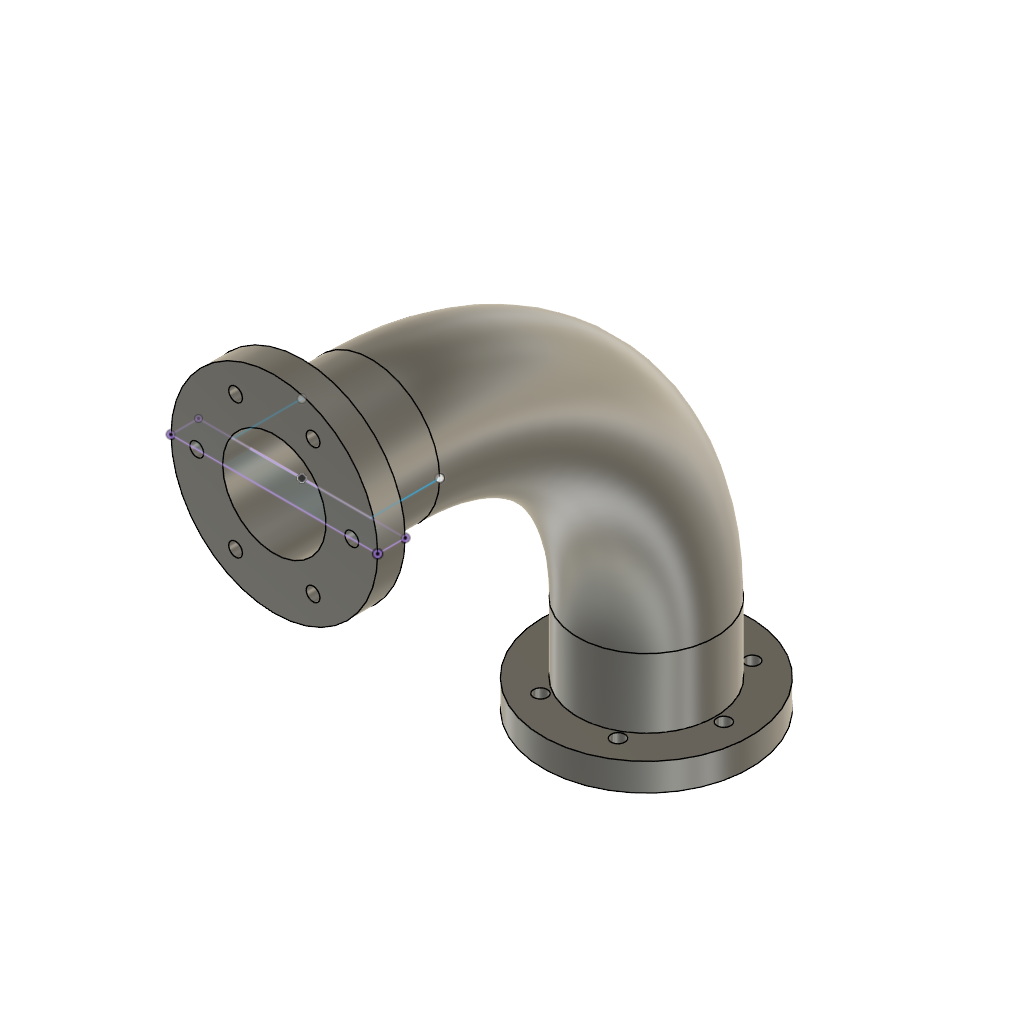
Exercise 1 (Autodesk Fusion 360 design; units mm, degrees)
part number: 2026-09-21-19-03-31-349
Autodesk Fusion 360 part; units mm, degrees
sketch "Sketch1" plane through (0, 0, 0) normal (0, 1, 0) x (1, 0, 0)
  circle A0 centre (0, 0) radius 37.5
  circle A1 centre (0, 0) radius 75
  line L0 (-75, 0) -> (-37.5, 0) construction
  circle A2 centre (-56.25, 0) radius 5
  line L1 (0, -75) -> (0, 75) construction
  circle A3 centre (56.25, 0) radius 5
  circle A4 centre (28.125, 48.7139) radius 5
  circle A5 centre (-28.125, 48.7139) radius 5
  circle A6 centre (-56.25, 0) radius 5
  circle A7 centre (-28.125, -48.7139) radius 5
  circle A8 centre (28.125, -48.7139) radius 5
  dimension "d1" = 75
  dimension "d2" = 150
  dimension "d3" = 10
  dimension "d5" = 360
  constraint coincident A0.centre A1.centre
  constraint concentric A0 A1
  constraint coincident A1 L0.start
  constraint coincident A0 L0.end
  constraint perpendicular A0 L0
  constraint midpoint L0 A2.centre
  constraint horizontal L0
  constraint coincident A1 L1.start
  constraint coincident A1 L1.end
  constraint perpendicular A1 L1
  constraint symmetric A2 L1 A3
  measures "d1" diameter of A0
  measures "d2" diameter of A1
  measures "d3" diameter of A2
extrude "Extrude1" add sketch "Sketch1" along normal blind 20
sketch "Sketch2" plane through (0, 0, 0) normal (0, 0, 1) x (1, 0, 0)
  line L0 (75, 20) -> (-75, 20)
  line L1 (-75, 0) -> (-75, 20)
  line L2 (75, 0) -> (-75, 0)
  line L3 (75, 0) -> (75, 20)
  line L4 (-50, 20) -> (50, 20)
  line L5 (-50, 20) -> (-50, 70)
  line L6 (50, 20) -> (50, 70)
  point P0 (0, 20)
  dimension "d8" = 100
  dimension "d9" = 50
  constraint midpoint L4 P0
  constraint coincident L0 P0
  constraint parallel L0 L4
  constraint perpendicular L4 L5
  constraint perpendicular L0 L6
  measures "d8" distance of L4.start L4.end
  measures "d9" distance of L4.start L5.end
sketch "Sketch3" plane through (0, 20, 0) normal (0, 1, 0) x (-1, 0, 0)
  circle A0 centre (28.125, 48.7139) radius 5
  circle A1 centre (-28.125, 48.7139) radius 5
  circle A2 centre (56.25, 0) radius 5
  circle A3 centre (0, 0) radius 37.5
  circle A4 centre (28.125, -48.7139) radius 5
  circle A5 centre (-56.25, 0) radius 5
  circle A6 centre (-28.125, -48.7139) radius 5
  circle A7 centre (0, 0) radius 75
  circle A8 centre (0, 0) radius 50
  dimension "d10" = 100
  constraint coincident A3.centre A7.centre
  measures "d10" diameter of A8
extrude "Extrude2" add sketch "Sketch3" along normal blind 50 contours A8
sketch "Sketch4" plane through (0, 70, 0) normal (0, 1, 0) x (-1, 0, 0)
  circle A0 centre (0, 0) radius 37.5
  circle A1 centre (0, 0) radius 50
sketch "Sketch5" plane through (0, 0, 0) normal (1, 0, 0) x (0, 1, 0)
  line L0 (70, -50) -> (70, 50)
  line L1 (20, 50) -> (70, 50)
  line L2 (20, 50) -> (20, 75)
  line L3 (0, 75) -> (20, 75)
  line L4 (0, 0) -> (0, 75)
  line L5 (0, -75) -> (0, 0)
  line L6 (0, -75) -> (20, -75)
  line L7 (20, -75) -> (20, -50)
  line L8 (20, -50) -> (70, -50)
  arc A0 (270, -200) -> (70, 0) centre (70, -200) ccw construction
  line L9 (20, 0) -> (70, 0)
  dimension "d13" = 200
  constraint midpoint L0 A0.end
  constraint tangent A0 L9
  measures "d13" radius of A0
sweep "Sweep1" add profiles "Sketch4" path "Sketch5" along A0 section 1
sketch "Sketch6" plane through (0, 0, -200) normal (0, 0, -1) x (1, 0, 0)
  circle A0 centre (0, -270) radius 37.5
  circle A1 centre (0, -270) radius 50
sketch "Sketch7" plane through (0, 0, 0) normal (0, 1, 0) x (1, 0, 0)
extrude "Extrude3" add sketch "Sketch6" along normal blind 50
sketch "Sketch8" plane through (0, 0, -250) normal (0, 0, -1) x (1, 0, 0)
  circle A0 centre (0, -270) radius 37.5
  circle A1 centre (0, -270) radius 50
  circle A2 centre (0, -270) radius 75
  line L0 (0, -270) -> (75, -270) construction
  circle A3 centre (56.25, -270) radius 5
  line L1 (0, -345) -> (0, -195) construction
  circle A4 centre (28.125, -221.2861) radius 5
  circle A5 centre (-28.125, -221.2861) radius 5
  circle A6 centre (-56.25, -270) radius 5
  circle A7 centre (-28.125, -318.7139) radius 5
  circle A8 centre (28.125, -318.7139) radius 5
  dimension "d23" = 150
  dimension "d24" = 10
  dimension "d25" = 56.25
  dimension "d27" = 360
  constraint concentric A0 A2
  constraint coincident A0.centre A1.centre
  constraint coincident A2 L0.end
  constraint horizontal L0
  constraint coincident L0 A3.centre
  constraint coincident A2 L1.start
  constraint coincident A2 L1.end
  constraint perpendicular A2 L1
  measures "d23" diameter of A2
  measures "d24" diameter of A3
  measures "d25" distance of A0.centre A3.centre
extrude "Extrude4" add sketch "Sketch8" along normal blind 20 contours A1 | A2
